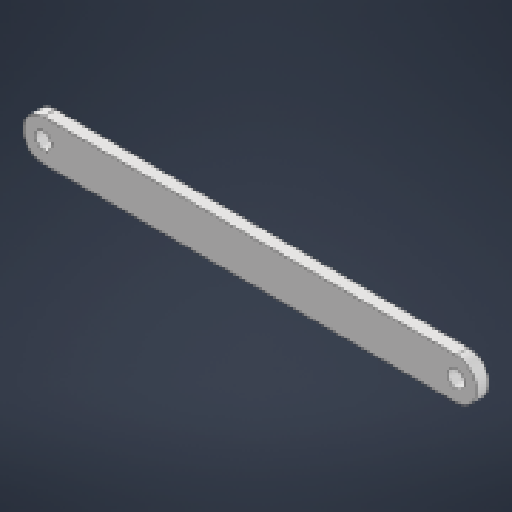
# Autodesk Inventor part: 连杆1
Saved by Autodesk Inventor 2025 (Build 290162000, 162)
## iProperties
Created: 2026-01-03
Part Number: 连杆1
Material: 常规
Document SubType Name: Modeling
Designer: XH
Density: 1 g/cm^3
Appearance: 默认
Author: XH
Autodesk Inventor part; units mm, degrees
ref_plane "YZ Plane" through (0, 0, 0) normal (1, 0, 0) x (0, 1, 0)
ref_plane "XZ Plane" through (0, 0, 0) normal (0, 1, 0) x (-1, 0, 0)
ref_plane "XY Plane" through (0, 0, 0) normal (0, 0, 1) x (1, 0, 0)
sketch "草图1" plane through (0, 0, 0) normal (0, 0, 1) x (1, 0, 0)
  line L0 (-50, 0) -> (50, 0) construction
  line L1 (-50, -5) -> (50, -5)
  line L2 (50, 5) -> (-50, 5)
  arc A0 (-50, 5) -> (-50, -5) centre (-50, 0) ccw
  arc A1 (50, -5) -> (50, 5) centre (50, 0) ccw
  point P0 (0, 0)
  dimension "d1" = 100
  dimension "d4" = 10
  constraints: 8 end point, 4 point on circle, 4 tangent, 2 centre point, 1 horizontal, 1 midpoint, 1 parallel
  measures "d1" distance of L0.start L0.end
  measures "d4" distance between parallel lines of L2 L1
extrude "拉伸1" add sketch "草图1" along normal blind 3
sketch "草图2" plane through (0, 0, 0) normal (0, 0, -1) x (-1, 0, 0)
  arc A0 (50, -5) -> (50, 5) centre (50, 0) ccw projected
  circle A1 centre (50, 0) radius 2
  line L0 (0, 0) -> (0, -18.0747)
  arc A2 (-50, 5) -> (-50, -5) centre (-50, 0) ccw
  circle A3 centre (-50, 0) radius 2
  dimension "d5" = 4
  constraints: 4 symmetric about line, 3 centre point, 2 coincident, 2 end point, 2 point on circle, 1 vertical, 2 other
  measures "d5" diameter of A1
extrude "拉伸2" cut sketch "草图2" against normal blind 10
